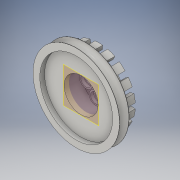
# Autodesk Inventor part: wheel
Saved by Autodesk Inventor 2016 (Build 200138000, 138)
## iProperties
Created: 2016-02-13
Part Number: wheel
Material: PC/ABS Plastic
Document SubType Name: Modeling
Designer: jforce
Density: 0.357273 g/cm^3
Appearance: Smooth - White
Author: jforce
## iProperties of the stored document wheel_3DPrint.ipt
Created: 2016-02-17
Part Number: wheel_3DPrint
Material: Generic
Document SubType Name: Modeling
Designer: jforce
Density: 1 g/cm^3
Appearance: Default
Author: jforce
Autodesk Inventor part; units mm, degrees
ref_plane "YZ Plane" through (0, 0, 0) normal (1, 0, 0) x (0, 1, 0)
ref_plane "XZ Plane" through (0, 0, 0) normal (0, 1, 0) x (-1, 0, 0)
ref_plane "XY Plane" through (0, 0, 0) normal (0, 0, 1) x (1, 0, 0)
sketch "Sketch1" plane through (0, 0, 0) normal (0, 0, 1) x (1, 0, 0)
  circle A0 centre (0, 0) radius 12
  dimension "d0" = 24
  constraints: 1 centre point, 1 coincident
  measures "d0" diameter of A0
extrude "Extrusion1" add sketch "Sketch1" along normal blind 3
sketch "Sketch2" plane through (0, 0, 3) normal (0, 0, 1) x (1, 0, 0)
  circle A0 centre (0, 0) radius 10.5
  circle A1 centre (0, 0) radius 12
  dimension "d3" = 21
  dimension "d4" = 24
  constraints: 2 centre point, 2 coincident
  measures "d3" diameter of A0
  measures "d4" diameter of A1
extrude "Extrusion2" add sketch "Sketch2" along normal blind 8
sketch "Sketch4" plane through (0, 0, 3) normal (0, 0, 1) x (1, 0, 0)
  line L0 (0, 0) -> (0, -6) construction
  dimension "d10" = 6
  constraints: 2 end point, 1 vertical
  measures "d10" distance of L0.start L0.end
hole "Hole1" at (0, -6, 3) direction (0, 0, -1) diameter 4 depth 3 tip angle 118 counterbore diameter 5 counterbore depth 0.85
pattern_circular "Circular Pattern1" count 4 over 360 about axis through (0, 0, -10) along (0, 0, 1) of "Hole1"
ref_plane "Work Plane1" through (0, 0, 14) normal (0, 0, 1) x (1, 0, 0)
sketch "Sketch5" plane through (0, 0, 14) normal (0, 0, 1) x (1, 0, 0)
  circle A0 centre (0, 0) radius 26.67
  circle A1 centre (0, 0) radius 22.5
  dimension "d21" = 45
  dimension "d35" = 53.34
  constraints: 2 centre point, 2 coincident
  measures "d21" diameter of A1
  measures "d35" diameter of A0
extrude "Extrusion4" add sketch "Sketch5" along normal blind 3
sketch "Sketch8" plane through (0, 0, 11) normal (0, 0, 1) x (1, 0, 0)
  circle A0 centre (0, 0) radius 10.5
  circle A1 centre (0, 0) radius 26.67
  dimension "d38" = 53.34
  constraints: 2 centre point, 2 coincident
  measures "d38" diameter of A1
extrude "Extrusion6" add sketch "Sketch8" along normal blind 3
sketch "Sketch6" plane through (0, 0, 0) normal (1, 0, 0) x (0, 1, 0)
  line L0 (-26.67, 11) -> (26.67, 11) projected
  line L1 (26.67, 17) -> (-26.67, 17) projected
  line L2 (0, -3.4) -> (0, 20.4) projected
  line L3 (-26.67, 14) -> (26.67, 14) projected
  circle A0 centre (26.67, 14) radius 2.8193
  point P0 (0, 0)
  point P1 (-22, 14)
  point P2 (-22.067, 14)
  constraints: 1 centre point, 1 coincident
revolve "Revolution1" cut sketch "Sketch6" angle 360 about axis through (0, 0, -10) along (0, 0, 1)
ref_plane "Work Plane2" through (0, 0, 11) normal (0, 0, -1) x (-1, 0, 0)
sketch "Sketch7" plane through (0, 0, 11) normal (0, 0, -1) x (-1, 0, 0)
  circle A0 centre (0, 0) radius 12 projected
  line L0 (0, 0) -> (29.1463, 0) construction
  line L1 (0, 0) -> (28.4807, 0) construction
  arc A1 (2.0864, 19.8507) -> (-2.0864, 19.8507) centre (0, 0) ccw
  arc A2 (2.3519, 22.3767) -> (-2.3519, 22.3767) centre (0, 0) ccw
  line L2 (-2.0864, 19.8507) -> (-2.3519, 22.3767)
  line L3 (2.0864, 19.8507) -> (2.3519, 22.3767)
  dimension "d28" = 45
  dimension "d41" = 2.54
  constraints: 8 end point, 4 point on circle, 2 centre point, 2 coincident, 2 horizontal
  measures "d28" diameter of A2
  measures "d41" radial gap between concentric circles of A1 A2
extrude "Extrusion5" add sketch "Sketch7" along normal blind 8 contours A1 L2 A2 L3
chamfer "Chamfer1" distance 1.5875 angle 45 2 edges at (0, 22.5, 11) (0, 19.96, 11)
pattern_circular "Circular Pattern3" count 18 over 360 about axis through (0, 0, -10) along (0, 0, 1) of "Extrusion5", "Chamfer1"
sketch "Sketch9" plane through (0, 0, 3) normal (0, 0, 1) x (1, 0, 0)
  circle A0 centre (0, 6) radius 2 projected
  circle A1 centre (0, 6) radius 3.2016
  circle A2 centre (0, 6) radius 4.062
  point P0 (0, 0)
  constraints: 2 centre point, 2 coincident
extrude "Extrusion7" add sketch "Sketch9" along normal blind 2 contours A2
pattern_circular "Circular Pattern4" count 4 over 360 about axis through (0, 0, -10) along (0, 0, 1) of "Extrusion7"
body "Solid1"
